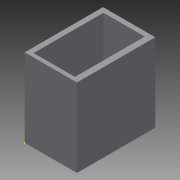
# Autodesk Inventor part: Part2
Saved by Autodesk Inventor 2015 (Build 190159000, 159)
## iProperties
Created: 2015-03-24
Part Number: Part2
Material: Generic
Document SubType Name: Modeling
Designer: nelsona
Density: 1 g/cm^3
Appearance: Default
Author: nelsona
Autodesk Inventor part; units mm, degrees
ref_plane "YZ Plane" through (0, 0, 0) normal (1, 0, 0) x (0, 1, 0)
ref_plane "XZ Plane" through (0, 0, 0) normal (0, 1, 0) x (-1, 0, 0)
ref_plane "XY Plane" through (0, 0, 0) normal (0, 0, 1) x (1, 0, 0)
sketch "Sketch1" plane through (0, 0, 0) normal (0, 1, 0) x (-1, 0, 0)
  line L0 (0, 0) -> (-50.8, 0)
  line L1 (-50.8, 0) -> (-50.8, -76.2)
  line L2 (-50.8, -76.2) -> (0, -76.2)
  line L3 (0, -76.2) -> (0, 0)
  line L4 (-4.0754, 0) -> (-4.0754, -6.35)
  line L5 (0, -6.35) -> (-6.35, -6.35)
  line L6 (-50.8, -76.2) -> (-50.8, -69.85)
  line L7 (-50.8, -69.85) -> (-44.45, -69.85)
  line L8 (-6.35, -6.35) -> (-44.45, -6.35)
  line L9 (-44.45, -6.35) -> (-44.45, -69.85)
  line L10 (-44.45, -69.85) -> (-6.35, -69.85)
  line L11 (-6.35, -69.85) -> (-6.35, -6.35)
  dimension "d0" = 50.8
  dimension "d1" = 76.2
  dimension "d2" = 6.35
  dimension "d3" = 6.35
  dimension "d4" = 6.35
  dimension "d5" = 6.35
  constraints: 24 end point, 4 parallel, 3 horizontal, 3 perpendicular, 3 point on line, 1 vertical
  measures "d0" distance of L2.end L1.end
  measures "d1" distance of L1.end L0.end
  measures "d2" distance of L4.start L4.end
  measures "d3" distance of L5.start L5.end
  measures "d4" distance of L1.end L6.end
  measures "d5" distance of L6.end L7.end
sketch "Sketch2" plane through (0, 0, 0) normal (0, 1, 0) x (-1, 0, 0)
  line L0 (-15.4991, -17.1025) -> (-35.8913, -17.1025)
  line L1 (-35.8913, -17.1025) -> (-35.8913, -58.0981)
  line L2 (-35.8913, -58.0981) -> (-15.4991, -58.0981)
  line L3 (-15.4991, -58.0981) -> (-15.4991, -17.1025)
  line L4 (-13.6908, -9.3345) -> (-8.6145, -9.1421)
  line L5 (-38.0829, -65.7666) -> (-42.7545, -67.7622)
  line L6 (-8.6145, -9.1421) -> (-42.7545, -9.1421)
  line L7 (-42.7545, -9.1421) -> (-42.7545, -67.7622)
  line L8 (-42.7545, -67.7622) -> (-8.6145, -67.7622)
  line L9 (-8.6145, -67.7622) -> (-8.6145, -9.1421)
  circle A0 centre (-20.5918, -13.1147) radius 1.651
  circle A1 centre (-30.7772, -13.1147) radius 1.651
  circle A2 centre (-20.5918, -62.0859) radius 1.651
  circle A3 centre (-30.7772, -62.0859) radius 1.651
  point P0 (0, 0)
  dimension "d6" = 40.9956
  dimension "d7" = 7.9756
  dimension "d8" = 5.08
  dimension "d9" = 7.9756
  dimension "d10" = 5.08
  dimension "d11" = 3.302
  dimension "d12" = 3.302
  dimension "d13" = 3.302
  dimension "d14" = 3.302
  dimension "d15" = 6.8846
  dimension "d16" = 6.8633
  constraints: 20 end point, 4 centre point, 4 parallel, 2 horizontal, 2 perpendicular
  measures "d6" distance of L1.end L0.end
  measures "d7" distance of L0.start L4.start
  measures "d8" distance of L4.start L4.end
  measures "d9" distance of L1.end L5.start
  measures "d10" distance of L5.start L5.end
  measures "d11" diameter of A0
  measures "d12" diameter of A1
  measures "d13" diameter of A2
  measures "d14" diameter of A3
  measures "d15" distance between parallel lines of L9 L3
  measures "d16" distance between parallel lines of L7 L1
sketch "Sketch3" plane through (0, 0, 0) normal (0, 1, 0) x (-1, 0, 0)
  line L0 (-6.35, -6.35) -> (-44.45, -6.35)
  line L1 (-44.45, -6.35) -> (-44.45, -69.85)
  line L2 (-44.45, -69.85) -> (-6.35, -69.85)
  line L3 (-6.35, -69.85) -> (-6.35, -6.35)
  point P0 (0, 0)
  constraints: 8 end point, 2 parallel, 1 horizontal, 1 perpendicular
extrude "Extrusion1" add sketch "Sketch1" along normal blind 76.2
sketch "Sketch4" plane through (0, 76.2, 0) normal (0, 1, 0) x (1, 0, 0)
  line L0 (45.1232, 71.603) -> (4.9996, 71.603)
  line L1 (4.9996, 71.603) -> (4.9996, 3.7205)
  line L2 (4.9996, 3.7205) -> (45.1232, 3.7205)
  line L3 (45.1232, 3.7205) -> (45.1232, 71.603)
  point P0 (0, 0)
  constraints: 8 end point, 3 perpendicular, 1 horizontal
extrude "Extrusion2" cut sketch "Sketch4" against normal blind 69.85
sketch "Sketch5" plane through (50.8, 0, -76.2) normal (0, 0, -1) x (-1, 0, 0)
  circle A0 centre (24.7613, 36.4788) radius 8.1657
  point P0 (50.8, 0)
  constraints: 1 centre point
extrude "Extrusion3" cut sketch "Sketch5" against normal blind 25.4
extrude "Extrusion4" cut sketch "Sketch2" along normal through all contours L3 L2 L1 L0 | A0 | A1 | A2 | A3
body "Solid1"
